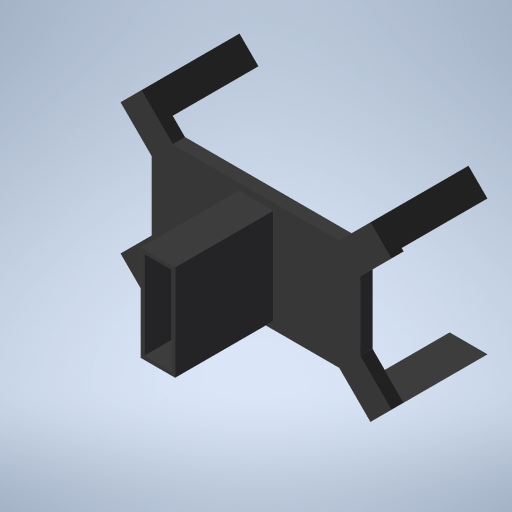
# Autodesk Inventor part: Part3
Saved by Autodesk Inventor 2024 (Build 280153000, 153)
## iProperties
Created: 2024-06-13
Part Number: Part3
Material: Generic
Document SubType Name: Sheet Metal
Designer: albah
Density: 1 g/cm^3
Sheet Metal Rule: Default_mm
Appearance: Default
Author: albah
Autodesk Inventor part; units mm, degrees
ref_plane "YZ Plane" through (0, 0, 0) normal (1, 0, 0) x (0, 1, 0)
ref_plane "XZ Plane" through (0, 0, 0) normal (0, 1, 0) x (-1, 0, 0)
ref_plane "XY Plane" through (0, 0, 0) normal (0, 0, 1) x (1, 0, 0)
sketch "Sketch1" plane through (0, 0, 0) normal (0, 0, 1) x (1, 0, 0)
  line L0 (0, 0) -> (85, 0)
  line L1 (85, 0) -> (85, -45)
  line L2 (85, -45) -> (0, -45)
  line L3 (0, -45) -> (0, 0)
  line L4 (0, -45) -> (-8.4853, -53.4853)
  line L5 (0, -45) -> (12, -45) construction
  line L6 (0, 0) -> (-8.4853, 8.4853)
  line L7 (0, 0) -> (12, 0) construction
  line L8 (85, 0) -> (93.4853, 8.4853)
  line L9 (85, 0) -> (97, 0) construction
  line L10 (85, -45) -> (93.4853, -53.4853)
  line L11 (-8.4853, 8.4853) -> (-4.2426, 12.7279)
  line L12 (-8.4853, 8.4853) -> (-12.7279, 4.2426)
  line L13 (93.4853, 8.4853) -> (89.2426, 12.7279)
  line L14 (93.4853, 8.4853) -> (97.7279, 4.2426)
  line L15 (93.4853, -53.4853) -> (97.7279, -49.2426)
  line L16 (93.4853, -53.4853) -> (89.2426, -57.7279)
  line L17 (-8.4853, -53.4853) -> (-4.2426, -57.7279)
  line L18 (-8.4853, -53.4853) -> (-12.7279, -49.2426)
  line L19 (-12.7279, -49.2426) -> (0, -36.5147)
  line L20 (-4.2426, -57.7279) -> (8.4853, -45)
  line L21 (-12.7279, 4.2426) -> (0, -8.4853)
  line L22 (-4.2426, 12.7279) -> (8.4853, 0)
  line L23 (89.2426, 12.7279) -> (76.5147, 0)
  line L24 (97.7279, 4.2426) -> (85, -8.4853)
  line L25 (97.7279, -49.2426) -> (85, -36.5147)
  line L26 (89.2426, -57.7279) -> (76.5147, -45)
  line L27 (-14.0147, 5.05) -> (99.0147, 5.05)
  line L28 (99.0147, 5.05) -> (99.0147, -50.05)
  line L29 (99.0147, -50.05) -> (-14.0147, -50.05)
  line L30 (-14.0147, -50.05) -> (-14.0147, 5.05)
  line L31 (-14.0147, 5.05) -> (99.0147, -50.05) construction
  line L32 (99.0147, 5.05) -> (-14.0147, -50.05) construction
  line L33 (37, -40.5) -> (48, -40.5)
  line L34 (48, -40.5) -> (48, -4.5)
  line L35 (48, -4.5) -> (37, -4.5)
  line L36 (37, -4.5) -> (37, -40.5)
  line L37 (37, -40.5) -> (48, -4.5) construction
  line L38 (48, -40.5) -> (37, -4.5) construction
  line L39 (49.5, -3) -> (35.5, -3)
  line L40 (35.5, -3) -> (35.5, -42)
  line L41 (35.5, -42) -> (49.5, -42)
  line L42 (49.5, -42) -> (49.5, -3)
  line L43 (49.5, -3) -> (35.5, -42) construction
  line L44 (35.5, -3) -> (49.5, -42) construction
  point P0 (42.5, -22.5)
  point P1 (96.9206, 5.05)
  point P2 (81.5647, 5.05)
  point P3 (81.5647, -50.05)
  point P4 (96.9206, -50.05)
  point P5 (-11.9206, -50.05)
  point P6 (3.4353, -50.05)
  point P7 (3.4353, 5.05)
  point P8 (-11.9206, 5.05)
  point P9 (8.4853, 0)
  dimension "d0" = 85
  dimension "d1" = 45
  dimension "d5" = 135
  dimension "d7" = 45
  dimension "d9" = 6
  dimension "d10" = 6
  dimension "d11" = 6
  dimension "d12" = 55.1
  dimension "d13" = 11
  dimension "d14" = 36
  dimension "d15" = 14
  dimension "d16" = 39
  constraints: 90 end point, 11 parallel, 8 point on line, 7 horizontal, 7 perpendicular, 6 midpoint, 3 equal length
  measures "d0" distance of L1.end L2.end
  measures "d1" distance of L0.end L1.end
  measures "d5" angle of L7 L6
  measures "d7" angle of L9 L8
  measures "d9" distance of L11.start L11.end
  measures "d10" distance of L11.start L12.end
  measures "d11" distance of L10.end L15.end
  measures "d12" distance of L27.end L28.end
  measures "d13" distance of L35.end L34.end
  measures "d14" distance of L34.end L33.end
  measures "d15" distance of L41.end L40.end
  measures "d16" distance of L40.end L39.end
extrude "Extrusion1" add sketch "Sketch1" against normal blind 5 contours L6 L27 L22 L0 | L0 L1 L2 L3 | L3 L21 L12 L27 L6 | L23 L27 L8 L0 | L3 L4 L29 L18 L19 | L8 L27 L14 L24 L1 | L2 L20 L29 L4 | L25 L15 L29 L10 L1 | L2 L10 L29 L26
extrude "Extrusion2" add sketch "Sketch1" against normal blind 40 contours L27 L12 L6 | L6 L11 L22 L27 | L23 L13 L8 L27 | L8 L14 L27 | L29 L20 L17 L4 | L4 L18 L29 | L29 L10 L16 L26 | L29 L15 L10
extrude "Extrusion3" add sketch "Sketch1" along normal blind 40 contours L42 L41 L40 L39
equation "\"BendRadius\" = Thickness"
equation "\"BendReliefWidth\" = Thickness"
equation "\"BendReliefDepth\" = 0.5 * Thickness"
equation "\"CornerReliefSize\" = 4 * Thickness"
equation "\"MinimumRemnant\" = 2 * Thickness"
equation "\"TransitionRadius\" = BendRadius"
equation "\"JacobiRadiusSize\" = BendRadius"
equation "\"GapSize\" = Thickness"
equation "\"Thickness\" = 0.5"
body "Solid1"
